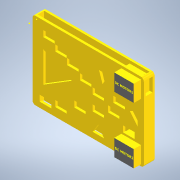
# Autodesk Inventor part: BASE7
Saved by Autodesk Inventor 2021 (Build 250183000, 183)
## iProperties
Created: 2021-07-07
Part Number: BASE7
Material: Generic
Document SubType Name: Modeling
Designer: AKSHATA
Density: 1 g/cm^3
Appearance: Glossy - Gold
Author: AKSHATA
Autodesk Inventor part; units mm, degrees
ref_plane "YZ Plane" through (0, 0, 0) normal (1, 0, 0) x (0, 1, 0)
ref_plane "XZ Plane" through (0, 0, 0) normal (0, 1, 0) x (-1, 0, 0)
ref_plane "XY Plane" through (0, 0, 0) normal (0, 0, 1) x (1, 0, 0)
sketch "Sketch1" plane through (0, 0, 0) normal (0, 0, 1) x (1, 0, 0)
  line L0 (-11.2354, 6.8902) -> (298.7646, 6.8902)
  line L1 (298.7646, 6.8902) -> (298.7646, -209.1098)
  line L2 (298.7646, -209.1098) -> (-11.2354, -209.1098)
  line L3 (-11.2354, -209.1098) -> (-11.2354, 6.8902)
  point P0 (0, 0)
  dimension "d0" = 310
  dimension "d1" = 216
  constraints: 8 end point, 2 parallel, 1 horizontal, 1 perpendicular
  measures "d0" distance of L1.end L2.end
  measures "d1" distance of L0.end L1.end
extrude "Extrusion1" add sketch "Sketch1" along normal blind 30
fillet "Fillet1" radius 8 4 edges at (298.7646, 6.8902, 15) (-11.2354, 6.8902, 15) (-11.2354, -209.1098, 15) (298.7646, -209.1098, 15)
sketch "Sketch2" plane through (-3.2354, 6.8902, 0) normal (0, 1, 0) x (1, 0, 0)
  line L0 (0, -30) -> (0, 0) projected
  line L1 (294, 0) -> (0, 0) projected
  point P0 (3.2354, 0)
  point P1 (15, -15)
  dimension "d5" = 15
  dimension "d6" = 15
  measures "d5" distance from line of L0 point (15, -15)
  measures "d6" distance from line of L1 point (15, -15)
hole "Hole1" at (11.7646, 6.8902, 15) direction (0, -1, 0) diameter 4 end through all
sketch "Sketch3" plane through (-3.2354, 6.8902, 0) normal (0, 1, 0) x (1, 0, 0)
  line L0 (294, 0) -> (294, -30) projected
  line L1 (294, 0) -> (0, 0) projected
  point P0 (3.2354, 0)
  point P1 (279, -15)
  dimension "d14" = 15
  dimension "d15" = 15
  measures "d14" distance from line of L0 point (279, -15)
  measures "d15" distance from line of L1 point (279, -15)
hole "Hole2" at (275.7646, 6.8902, 15) direction (0, -1, 0) diameter 4 end through all
sketch "Sketch4" plane through (-3.2354, -209.1098, 0) normal (0, -1, 0) x (1, 0, 0)
  line L0 (0, 30) -> (0, 0) projected
  line L1 (294, 30) -> (294, 0) projected
  line L2 (0, 23.4652) -> (294, 23.4652)
  line L3 (294, 23.4652) -> (294, 5.9445)
  line L4 (294, 5.9445) -> (0, 5.9445)
  line L5 (0, 5.9445) -> (0, 23.4652)
  point P0 (3.2354, 0)
  constraints: 8 end point, 2 parallel, 2 point on line, 1 horizontal, 1 perpendicular
extrude "Extrusion2" cut sketch "Sketch4" against normal blind 230
sketch "Sketch5" plane through (0, 0, 30) normal (0, 0, 1) x (1, 0, 0)
  line L0 (18.7722, -16.5821) -> (50.6849, -16.5821)
  line L1 (50.6849, -16.5821) -> (50.6849, -33.4771)
  line L2 (50.6849, -33.4771) -> (18.7722, -33.4771)
  line L3 (18.7722, -33.4771) -> (18.7722, -16.5821)
  line L4 (51.9364, -34.7285) -> (83.8491, -34.7285)
  line L5 (83.8491, -34.7285) -> (83.8491, -51.6235)
  line L6 (83.8491, -51.6235) -> (51.9364, -51.6235)
  line L7 (51.9364, -51.6235) -> (51.9364, -34.7285)
  line L8 (85.1006, -50.9978) -> (117.0133, -50.9978)
  line L9 (117.0133, -50.9978) -> (117.0133, -67.8927)
  line L10 (117.0133, -67.8927) -> (85.1006, -67.8927)
  line L11 (85.1006, -67.8927) -> (85.1006, -50.9978)
  line L12 (120.7677, -69.77) -> (152.6805, -69.77)
  line L13 (152.6805, -69.77) -> (152.6805, -86.6649)
  line L14 (152.6805, -86.6649) -> (120.7677, -86.6649)
  line L15 (120.7677, -86.6649) -> (120.7677, -69.77)
  line L16 (155.8092, -86.0392) -> (187.7219, -86.0392)
  line L17 (187.7219, -86.0392) -> (187.7219, -102.9342)
  line L18 (187.7219, -102.9342) -> (155.8092, -102.9342)
  line L19 (155.8092, -102.9342) -> (155.8092, -86.0392)
  line L20 (198.9852, -107.9401) -> (230.8979, -107.9401)
  line L21 (230.8979, -107.9401) -> (230.8979, -124.8351)
  line L22 (230.8979, -124.8351) -> (198.9852, -124.8351)
  line L23 (198.9852, -124.8351) -> (198.9852, -107.9401)
  line L24 (240.9097, -135.4726) -> (272.8225, -135.4726)
  line L25 (272.8225, -135.4726) -> (272.8225, -152.3676)
  line L26 (272.8225, -152.3676) -> (240.9097, -152.3676)
  line L27 (240.9097, -152.3676) -> (240.9097, -135.4726)
  line L28 (258.4305, -160.1893) -> (290.3432, -160.1893)
  line L29 (290.3432, -160.1893) -> (290.3432, -177.0843)
  line L30 (290.3432, -177.0843) -> (258.4305, -177.0843)
  line L31 (258.4305, -177.0843) -> (258.4305, -160.1893)
  line L32 (214.0029, -77.5917) -> (245.9157, -77.5917)
  line L33 (245.9157, -77.5917) -> (245.9157, -94.4867)
  line L34 (245.9157, -94.4867) -> (214.0029, -94.4867)
  line L35 (214.0029, -94.4867) -> (214.0029, -77.5917)
  line L36 (236.5296, -42.5503) -> (268.4423, -42.5503)
  line L37 (268.4423, -42.5503) -> (268.4423, -59.4453)
  line L38 (268.4423, -59.4453) -> (236.5296, -59.4453)
  line L39 (236.5296, -59.4453) -> (236.5296, -42.5503)
  line L40 (252.4859, -8.1346) -> (284.3987, -8.1346)
  line L41 (284.3987, -8.1346) -> (284.3987, -25.0296)
  line L42 (284.3987, -25.0296) -> (252.4859, -25.0296)
  line L43 (252.4859, -25.0296) -> (252.4859, -8.1346)
  line L44 (155.8092, -127.0251) -> (187.7219, -127.0251)
  line L45 (187.7219, -127.0251) -> (187.7219, -143.9201)
  line L46 (187.7219, -143.9201) -> (155.8092, -143.9201)
  line L47 (155.8092, -143.9201) -> (155.8092, -127.0251)
  line L48 (104.8114, -143.2944) -> (136.7241, -143.2944)
  line L49 (136.7241, -143.2944) -> (136.7241, -160.1893)
  line L50 (136.7241, -160.1893) -> (104.8114, -160.1893)
  line L51 (104.8114, -160.1893) -> (104.8114, -143.2944)
  line L52 (51.9364, -168.6368) -> (83.8491, -168.6368)
  line L53 (83.8491, -168.6368) -> (83.8491, -185.5318)
  line L54 (83.8491, -185.5318) -> (51.9364, -185.5318)
  line L55 (51.9364, -185.5318) -> (51.9364, -168.6368)
  line L56 (8.7604, -177.3972) -> (40.6731, -177.3972)
  line L57 (40.6731, -177.3972) -> (40.6731, -194.2922)
  line L58 (40.6731, -194.2922) -> (8.7604, -194.2922)
  line L59 (8.7604, -194.2922) -> (8.7604, -177.3972)
  point P0 (0, 0)
  constraints: 120 end point, 30 parallel, 15 horizontal, 15 perpendicular
extrude "Extrusion3" cut sketch "Sketch5" against normal blind 10
sketch "Sketch6" plane through (0, 0, 30) normal (0, 0, 1) x (1, 0, 0)
  line L0 (18.3995, -62.6662) -> (18.3995, -148.4751)
  line L1 (18.3995, -62.6662) -> (97.8638, -99.3877)
  line L2 (97.8638, -99.3877) -> (18.3995, -148.4751)
  line L3 (173.9608, -35.3426) -> (201.5422, -35.3426)
  line L4 (201.5422, -35.3426) -> (183.641, -64.3216)
  line L5 (183.641, -64.3216) -> (173.9608, -35.3426)
  line L6 (155.8092, -193.1916) -> (187.7219, -193.1916)
  line L7 (187.7219, -193.1916) -> (171.7655, -167.3609)
  line L8 (171.7655, -167.3609) -> (155.8092, -193.1916)
  line L9 (281.0984, -81.0269) -> (281.0984, -117.6665)
  line L10 (281.0984, -117.6665) -> (259.5106, -91.1698)
  line L11 (259.5106, -91.1698) -> (281.0984, -81.0269)
  point P0 (0, 0)
  constraints: 24 end point, 2 horizontal, 2 vertical, 1 parallel, 1 perpendicular, 1 point on line
extrude "Extrusion4" cut sketch "Sketch6" against normal blind 10
sketch "Sketch7" plane through (298.7646, -201.1098, 0) normal (1, 0, 0) x (0, 0, -1)
  line L0 (0, 200) -> (-30, 200) projected
  line L1 (-5.9445, -8) -> (-5.9445, 208) projected
  line L2 (-24.584, 200) -> (-5.9445, 200)
  line L3 (-5.9445, 200) -> (-5.9445, 162.1585)
  line L4 (-5.9445, 162.1585) -> (-24.584, 162.1585)
  line L5 (-24.584, 162.1585) -> (-24.584, 200)
  point P0 (0, 201.1098)
  constraints: 8 end point, 2 parallel, 2 point on line, 1 horizontal, 1 perpendicular
extrude "Extrusion5" cut sketch "Sketch7" against normal blind 50
sketch "Sketch8" plane through (0, 0, 30) normal (0, 0, 1) x (1, 0, 0)
  point P0 (0, 0)
sketch "Sketch9" plane through (0, 0, 30) normal (0, 0, 1) x (1, 0, 0)
  line L0 (290.7646, -209.1098) -> (290.7646, -38.9513) projected
  line L1 (236.1444, -157.8413) -> (290.7646, -157.8413)
  line L2 (290.7646, -157.8413) -> (290.7646, -204.3612)
  line L3 (290.7646, -204.3612) -> (236.1444, -204.3612)
  line L4 (236.1444, -204.3612) -> (236.1444, -157.8413)
  line L5 (236.1444, 0) -> (290.7646, 0)
  line L6 (290.7646, 0) -> (290.7646, -46.5198)
  line L7 (290.7646, -46.5198) -> (236.1444, -46.5198)
  line L8 (236.1444, -46.5198) -> (236.1444, 0)
  point P0 (0, 0)
  constraints: 16 end point, 4 parallel, 2 horizontal, 2 perpendicular, 1 point on line
extrude "Extrusion6" add sketch "Sketch9" along normal blind 20 and the other way blind 23
sketch "Sketch10" plane through (0, 0, 50) normal (0, 0, 1) x (1, 0, 0)
  line L0 (237.4967, -19.8194) -> (288.8919, -19.8194) construction
  line L1 (288.8919, -19.8194) -> (288.8919, -26.1765) construction
  line L2 (288.8919, -26.1765) -> (237.4967, -26.1765) construction
  line L3 (237.4967, -26.1765) -> (237.4967, -19.8194) construction
  line L4 (237.994, -177.8514) -> (289.3892, -177.8514) construction
  line L5 (289.3892, -177.8514) -> (289.3892, -184.2084) construction
  line L6 (289.3892, -184.2084) -> (237.994, -184.2084) construction
  line L7 (237.994, -184.2084) -> (237.994, -177.8514) construction
  point P0 (0, 0)
  dimension "d0" = 310
  dimension "d1" = 216
  constraints: 4 other
sketch "Sketch11" plane through (236.1444, 0, 23.4652) normal (0, 1, 0) x (1, 0, 0)
  circle A0 centre (48.3692, 10.3631) radius 2.0886
  point P0 (-236.1444, 23.4652)
  constraints: 1 centre point
extrude "Extrusion7" cut sketch "Sketch11" against normal blind 220
sketch "Sketch12" plane through (-3.2354, 6.8902, 30) normal (0, 1, 0) x (1, 0, 0)
  line L0 (0, 6.5348) -> (0, 24.0555) projected
  line L1 (294, 24.0555) -> (0, 24.0555) projected
  line L2 (0, 6.5348) -> (43.8281, 6.5348)
  line L3 (43.8281, 6.5348) -> (43.8281, 24.0555)
  line L4 (43.8281, 24.0555) -> (0, 24.0555)
  line L5 (0, 24.0555) -> (0, 6.5348)
  point P0 (3.2354, 30)
  constraints: 8 end point, 2 parallel, 1 horizontal, 1 perpendicular, 1 point on line
extrude "Extrusion8" add sketch "Sketch12" against normal blind 216
sketch "Sketch13" plane through (-3.2354, 6.8902, 0) normal (0, 1, 0) x (1, 0, 0)
  circle A0 centre (16.9989, -11.4695) radius 6.0425
  point P0 (3.2354, 0)
  constraints: 1 centre point
extrude "Extrusion9" cut sketch "Sketch13" against normal blind 216
body "Solid1"
